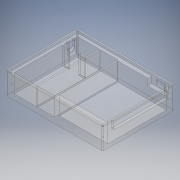
# Autodesk Inventor part: Fond boitier
Saved by Autodesk Inventor 2018.1 (Build 221171000, 171)
## iProperties
Created: 2024-08-14
Part Number: Fond boitier
Material: PET Plastic
Document SubType Name: Modeling
Designer: mouta
Density: 1.541 g/cm^3
Appearance: Polycarbonate - Clear
Mass: 547.24 g
Surface Area: 1254.22 cm^2
Volume: 355.12 cm^3
Author: mouta
Autodesk Inventor part; units mm, degrees
ref_plane "YZ Plane" through (0, 0, 0) normal (1, 0, 0) x (0, 1, 0)
ref_plane "XZ Plane" through (0, 0, 0) normal (0, 1, 0) x (-1, 0, 0)
ref_plane "XY Plane" through (0, 0, 0) normal (0, 0, 1) x (1, 0, 0)
sketch "Fond" plane through (0, 0, 0) normal (0, 0, 1) x (1, 0, 0)
  line L0 (2, 0) -> (188, 0)
  line L1 (190, 2) -> (190, 138)
  line L2 (188, 140) -> (2, 140)
  line L3 (0, 138) -> (0, 2)
  arc A0 (2, 140) -> (0, 138) centre (2, 138) ccw
  arc A1 (190, 138) -> (188, 140) centre (188, 138) ccw
  arc A2 (188, 0) -> (190, 2) centre (188, 2) ccw
  arc A3 (0, 2) -> (2, 0) centre (2, 2) ccw
  point P0 (0, 0)
  point P1 (190, 140)
  point P2 (190, 0)
  point P3 (0, 140)
  dimension "d0" = 190
  dimension "d1" = 140
  dimension "d2" = 2
  constraints: 8 end point, 8 point on circle, 8 point on line, 8 tangent, 4 centre point, 3 equal radius, 2 parallel, 1 horizontal, 1 perpendicular
  measures "d0" distance of point (0, 140) point (190, 140)
  measures "d1" distance of point (190, 140) point (190, 0)
  measures "d2" radius of A0
extrude "Extrusion1" add sketch "Fond" along normal blind 3
sketch "Sketch2" plane through (0, 0, 3) normal (0, 0, 1) x (1, 0, 0)
  line L0 (2, 0) -> (188, 0)
  line L1 (190, 2) -> (190, 138)
  line L2 (188, 140) -> (2, 140)
  line L3 (0, 138) -> (0, 2)
  arc A0 (190, 138) -> (188, 140) centre (188, 138) ccw
  arc A1 (188, 0) -> (190, 2) centre (188, 2) ccw
  arc A2 (0, 2) -> (2, 0) centre (2, 2) ccw
  arc A3 (2, 140) -> (0, 138) centre (2, 138) ccw
  line L4 (185, 130) -> (185, 15)
  line L5 (90, 130) -> (90, 15)
  line L6 (90, 130) -> (185, 130)
  line L7 (90, 15) -> (185, 15)
  line L8 (51, 8) -> (51, 15)
  line L9 (87, 132) -> (87, 8)
  line L10 (8, 8) -> (8, 103)
  line L11 (54, 103) -> (54, 110)
  line L12 (87, 132) -> (54, 132)
  line L13 (54, 103) -> (54, 8)
  line L14 (51, 103) -> (51, 8)
  line L15 (54, 103) -> (54, 132)
  line L16 (87, 8) -> (54, 8)
  line L17 (51, 8) -> (8, 8)
  line L18 (51, 106) -> (51, 132)
  line L19 (51, 132) -> (8, 132)
  line L20 (8, 132) -> (8, 106)
  line L21 (8, 103) -> (19.5, 103)
  line L22 (39.5, 103) -> (39.5, 106)
  line L23 (19.5, 103) -> (19.5, 106)
  line L24 (8, 106) -> (19.5, 106)
  line L25 (39.5, 106) -> (51, 106)
  line L26 (8, 103) -> (19.5, 103)
  line L27 (39.5, 103) -> (51, 103)
  point P0 (0, 0)
  dimension "d5" = 2
  dimension "d15" = 3
  dimension "d63" = 115
  dimension "d64" = 15
  constraints: 56 end point, 16 perpendicular, 8 point on circle, 8 tangent, 4 centre point, 3 equal radius, 3 parallel, 3 point on line, 1 horizontal, 1 vertical
  measures "d5" radius of A0
  measures "d15" distance between parallel lines of L5 L9
  measures "d63" distance between parallel lines of L7 L6
  measures "d64" distance between parallel lines of L0 L7
extrude "Extrusion2" add sketch "Sketch2" along normal blind 36
sketch "Sketch3" plane through (0, 0, 39) normal (0, 0, 1) x (1, 0, 0)
  line L0 (2, 0) -> (188, 0)
  line L1 (190, 2) -> (190, 138)
  line L2 (188, 140) -> (2, 140)
  line L3 (0, 138) -> (0, 2)
  arc A0 (190, 138) -> (188, 140) centre (188, 138) ccw
  arc A1 (188, 0) -> (190, 2) centre (188, 2) ccw
  arc A2 (0, 2) -> (2, 0) centre (2, 2) ccw
  arc A3 (2, 140) -> (0, 138) centre (2, 138) ccw
  line L4 (2.5, 137.5) -> (187.5, 137.5)
  line L5 (187.5, 137.5) -> (187.5, 2.5)
  line L6 (187.5, 2.5) -> (2.5, 2.5)
  line L7 (2.5, 2.5) -> (2.5, 137.5)
  point P0 (0, 0)
  dimension "d23" = 2
  dimension "d24" = 2.5
  constraints: 16 end point, 8 point on circle, 8 tangent, 4 centre point, 4 parallel, 3 equal radius, 2 perpendicular, 2 point on line, 1 horizontal, 3 other
  measures "d23" radius of A0
  measures "d24" distance between parallel lines of L2 L4
extrude "Extrusion3" add sketch "Sketch3" along normal blind 5
hole "Hole1" at (185, 135, 39) direction (0, 0, -1) diameter 3 depth 20 tip angle 118
hole "Hole2" at (185, 5, 39) direction (0, 0, -1) diameter 3 depth 20 tip angle 118
hole "Hole3" at (5, 5, 39) direction (0, 0, -1) diameter 3 depth 20 tip angle 118
hole "Hole4" at (5, 135, 39) direction (0, 0, -1) diameter 3 depth 20 tip angle 118
sketch "Sketch4" plane through (190, 2, 0) normal (1, 0, 0) x (0, 0, -1)
  line L0 (-3, 13) -> (-39, 13) projected
  line L1 (-3, 128) -> (-39, 128) projected
  line L2 (-26.7568, 124.9888) -> (-14.5206, 124.9888) construction
  line L3 (-39, 13) -> (-39, 20)
  line L4 (-39, 21) -> (-39, 124)
  line L5 (-38, 125) -> (-26.5, 125)
  line L6 (-25.5, 124) -> (-25.5, 21)
  line L7 (-26.5, 20) -> (-38, 20)
  arc A0 (-39, 21) -> (-38, 20) centre (-38, 21) ccw
  arc A1 (-26.5, 20) -> (-25.5, 21) centre (-26.5, 21) ccw
  arc A2 (-25.5, 124) -> (-26.5, 125) centre (-26.5, 124) ccw
  arc A3 (-38, 125) -> (-39, 124) centre (-38, 124) ccw
  point P0 (0, -2)
  point P1 (-41, 20.0871)
  point P2 (-39, 125)
  point P3 (-25.5, 125)
  dimension "d71" = 105
  dimension "d72" = 13.5
  dimension "d73" = 1
  constraints: 12 end point, 8 point on circle, 8 tangent, 6 point on line, 4 centre point, 3 equal radius, 2 perpendicular, 1 horizontal, 1 vertical
  measures "d71" distance of L3.end point (-39, 125)
  measures "d72" distance of point (-39, 125) point (-25.5, 125)
  measures "d73" radius of A0
extrude "Extrusion4" cut sketch "Sketch4" against normal blind 5
sketch "Sketch5" plane through (90, 130, 3) normal (0, -1, 0) x (1, 0, 0)
  line L0 (0, 36) -> (95, 36) projected
  line L1 (92, 36) -> (59, 36)
  line L2 (59, 36) -> (59, 23)
  line L3 (59, 23) -> (92, 23)
  line L4 (92, 23) -> (92, 36)
  point P0 (-90, -3)
  dimension "d76" = 33
  dimension "d77" = 13
  constraints: 8 end point, 2 parallel, 1 horizontal, 1 perpendicular, 1 point on line
  measures "d76" distance of L3.end L2.end
  measures "d77" distance of L2.end L1.end
extrude "Extrusion5" cut sketch "Sketch5" against normal blind 7.5
sketch "Sketch6" plane through (2.5, 137.5, 44) normal (0, -1, 0) x (1, 0, 0)
  line L0 (171, -7.5) -> (155, -7.5)
  line L1 (155, -7.5) -> (155, -15.5)
  line L2 (155, -15.5) -> (171, -15.5)
  line L3 (171, -15.5) -> (171, -7.5)
  point P0 (-2.5, -44)
  dimension "d80" = 16
  dimension "d81" = 8
  constraints: 8 end point, 2 parallel, 1 horizontal, 1 perpendicular
  measures "d80" distance of L2.end L1.end
  measures "d81" distance of L1.end L0.end
extrude "Extrusion6" cut sketch "Sketch6" against normal blind 7.5
sketch "Sketch7" plane through (0, 2, 0) normal (-1, 0, 0) x (0, 0, 1)
  line L0 (21, 128) -> (30, 128)
  line L1 (36, 122) -> (36, 122)
  line L2 (30, 116) -> (21, 116)
  line L3 (15, 122) -> (15, 122)
  line L4 (0, 136) -> (0, 0) projected
  arc A0 (21, 128) -> (15, 122) centre (21, 122) ccw
  arc A1 (15, 122) -> (21, 116) centre (21, 122) ccw
  arc A2 (30, 116) -> (36, 122) centre (30, 122) ccw
  arc A3 (36, 122) -> (30, 128) centre (30, 122) ccw
  point P0 (0, -2)
  point P1 (36, 116)
  point P2 (36, 128)
  point P3 (15, 116)
  dimension "d84" = 21
  dimension "d85" = 12
  dimension "d86" = 15
  dimension "d87" = 6
  constraints: 8 end point, 8 point on circle, 8 tangent, 6 point on line, 4 centre point, 3 equal radius, 2 parallel, 1 horizontal, 1 perpendicular
  measures "d84" distance of point (36, 116) point (15, 116)
  measures "d85" distance of point (36, 128) point (36, 116)
  measures "d86" distance between parallel lines of L4 L3
  measures "d87" radius of A0
extrude "Extrusion7" cut sketch "Sketch7" against normal blind 10
sketch "Sketch8" plane through (8, 106, 3) normal (1, 0, 0) x (0, 0, -1)
  line L0 (-32, 25) -> (-9, 25)
  line L1 (-9, 25) -> (-9, 11)
  line L2 (-9, 11) -> (-32, 11)
  line L3 (-32, 11) -> (-32, 25)
  point P0 (3, -106)
  dimension "d90" = 23
  dimension "d91" = 14
  constraints: 8 end point, 2 parallel, 1 horizontal, 1 perpendicular
  measures "d90" distance of L1.end L2.end
  measures "d91" distance of L0.end L1.end
extrude "Extrusion8" cut sketch "Sketch8" against normal blind 4
body "Solid1"
